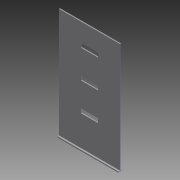
# Autodesk Inventor part: feederStationSlots
Saved by Autodesk Inventor 2011 SP1 (Build 150282100, 282)
## iProperties
Created: 2013-01-18
Part Number: feederStationSlots
Document SubType Name: Modeling
Designer: wes
Density: 1 g/cm^3
Author: wes
Autodesk Inventor part; units mm, degrees
ref_plane "YZ Plane" through (0, 0, 0) normal (1, 0, 0) x (0, 1, 0)
ref_plane "XZ Plane" through (0, 0, 0) normal (0, 1, 0) x (-1, 0, 0)
ref_plane "XY Plane" through (0, 0, 0) normal (0, 0, 1) x (1, 0, 0)
sketch "Sketch1" plane through (0, 0, 0) normal (0, 0, 1) x (1, 0, 0)
  line L0 (-140.3442, -2139.338) -> (951.8558, -2139.338)
  line L1 (951.8558, -2139.338) -> (951.8558, -158.138)
  line L2 (951.8558, -158.138) -> (-140.3442, -158.138)
  line L3 (-140.3442, -158.138) -> (-140.3442, -2139.338)
  line L4 (253.3558, -488.338) -> (558.1558, -488.338)
  line L5 (558.1558, -488.338) -> (558.1558, -564.538)
  line L6 (558.1558, -564.538) -> (253.3558, -564.538)
  line L7 (253.3558, -564.538) -> (253.3558, -488.338)
  line L8 (253.3558, -996.338) -> (558.1558, -996.338)
  line L9 (558.1558, -996.338) -> (558.1558, -1072.538)
  line L10 (558.1558, -1072.538) -> (253.3558, -1072.538)
  line L11 (253.3558, -1072.538) -> (253.3558, -996.338)
  line L12 (253.3558, -1504.338) -> (558.1558, -1504.338)
  line L13 (558.1558, -1504.338) -> (558.1558, -1580.538)
  line L14 (558.1558, -1580.538) -> (253.3558, -1580.538)
  line L15 (253.3558, -1580.538) -> (253.3558, -1504.338)
  point P0 (0, 0)
  dimension "d0" = 1092.2
  dimension "d1" = 1981.2
  dimension "d2" = 393.7
  dimension "d3" = 393.7
  dimension "d4" = 393.7
  dimension "d5" = 304.8
  dimension "d6" = 304.8
  dimension "d7" = 304.8
  dimension "d8" = 76.2
  dimension "d9" = 76.2
  dimension "d10" = 76.2
  dimension "d11" = 558.8
  dimension "d12" = 1066.8
  dimension "d13" = 1574.8
  constraints: 32 end point, 8 parallel, 4 horizontal, 4 perpendicular
  measures "d0" distance of L1.end L2.end
  measures "d1" distance of L2.end L0.start
  measures "d2" distance between parallel lines of L3 L7
  measures "d3" distance between parallel lines of L3 L11
  measures "d4" distance between parallel lines of L3 L15
  measures "d5" distance of L4.start L4.end
  measures "d6" distance of L8.start L8.end
  measures "d7" distance of L12.start L12.end
  measures "d8" distance of L4.end L5.end
  measures "d9" distance of L8.end L9.end
  measures "d10" distance of L12.end L13.end
  measures "d11" distance between parallel lines of L0 L14
  measures "d12" distance between parallel lines of L0 L10
  measures "d13" distance between parallel lines of L0 L6
extrude "Extrusion1" add sketch "Sketch1" against normal blind 19.05
sketch "Sketch2" plane through (-140.3442, -2139.338, 0) normal (0, -1, 0) x (1, 0, 0)
  line L0 (0, -19.05) -> (1092.2, -19.05) projected
  line L1 (1092.2, 0) -> (1092.2, -19.05) projected
  line L2 (0, 0) -> (1092.2, 0) projected
  line L3 (0, 0) -> (0, -19.05) projected
  line L4 (0, -19.05) -> (1092.2, -19.05) projected
  line L5 (1092.2, 0) -> (1092.2, -19.05) projected
  line L6 (0, 0) -> (1092.2, 0) projected
  line L7 (0, 0) -> (0, -19.05) projected
  line L8 (1092.2, 28.575) -> (0, 28.575)
  line L9 (0, 28.575) -> (0, -47.625)
  line L10 (0, -47.625) -> (1092.2, -47.625)
  line L11 (1092.2, -47.625) -> (1092.2, 28.575)
  point P0 (140.3442, 0)
  dimension "d16" = 76.2
  dimension "d17" = 28.575
  constraints: 8 end point, 2 parallel, 1 horizontal, 1 perpendicular
  measures "d16" distance of L10.end L8.start
  measures "d17" distance between parallel lines of L8 L2
extrude "Extrusion2" add sketch "Sketch2" against normal blind 19.05 contours L0 L11 L10 L9 | L9 L8 L11 L2
sketch "Sketch3" plane through (0, 0, -19.05) normal (0, 0, -1) x (-1, 0, 0)
  line L0 (-253.3558, -996.338) -> (-253.3558, -1072.538) projected
  line L1 (-253.3558, -1072.538) -> (-558.1558, -1072.538) projected
  line L2 (-558.1558, -1072.538) -> (-558.1558, -996.338) projected
  line L3 (-253.3558, -488.338) -> (-253.3558, -564.538) projected
  line L4 (-253.3558, -564.538) -> (-558.1558, -564.538) projected
  line L5 (-558.1558, -564.538) -> (-558.1558, -488.338) projected
  line L6 (-253.3558, -1504.338) -> (-253.3558, -1580.538) projected
  line L7 (-253.3558, -1580.538) -> (-558.1558, -1580.538) projected
  line L8 (-558.1558, -1580.538) -> (-558.1558, -1504.338) projected
  point P0 (0, 0)
  point P1 (-507.3558, -589.938)
  point P2 (-304.1558, -589.938)
  point P3 (-507.3558, -1097.938)
  point P4 (-304.1558, -1097.938)
  point P5 (-507.3558, -1605.938)
  point P6 (-304.1558, -1605.938)
  dimension "d20" = 50.8
  dimension "d21" = 50.8
  dimension "d22" = 25.4
  dimension "d23" = 25.4
  dimension "d24" = 50.8
  dimension "d25" = 50.8
  dimension "d26" = 25.4
  dimension "d27" = 25.4
  dimension "d28" = 50.8
  dimension "d29" = 25.4
  dimension "d30" = 50.8
  dimension "d31" = 25.4
  measures "d20" distance from line of point (-507.356, -589.938) L5
  measures "d21" distance from line of point (-304.156, -589.938) L3
  measures "d22" distance from line of point (-304.156, -589.938) L4
  measures "d23" distance from line of L4 point (-507.356, -589.938)
  measures "d24" distance from line of L2 point (-507.356, -1097.938)
  measures "d25" distance from line of L0 point (-304.156, -1097.938)
  measures "d26" distance from line of point (-304.156, -1097.938) L1
  measures "d27" distance from line of L1 point (-507.356, -1097.938)
  measures "d28" distance from line of point (-507.356, -1605.938) L8
  measures "d29" distance from line of L7 point (-507.356, -1605.938)
  measures "d30" distance from line of L6 point (-304.156, -1605.938)
  measures "d31" distance from line of L7 point (-304.156, -1605.938)
hole "Hole1" at (507.3558, -589.938, -19.05) at (304.1558, -589.938, -19.05) at (507.3558, -1097.938, -19.05) at (304.1558, -1097.938, -19.05) at (507.3558, -1605.938, -19.05) at (304.1558, -1605.938, -19.05) direction (0, 0, 1) diameter 6.858 depth 25.4 tip angle 118
thread "Thread1" size "5/16-18 UNC" class "2B" standard "ANSI Unified Screw Threads" full length
thread "Thread2" size "5/16-18 UNC" class "2B" standard "ANSI Unified Screw Threads" full length
thread "Thread3" size "5/16-18 UNC" class "2B" standard "ANSI Unified Screw Threads" full length
thread "Thread4" size "5/16-18 UNC" class "2B" standard "ANSI Unified Screw Threads" full length
thread "Thread5" size "5/16-18 UNC" class "2B" standard "ANSI Unified Screw Threads" full length
thread "Thread6" size "5/16-18 UNC" class "2B" standard "ANSI Unified Screw Threads" full length
equation "\"d6\" = d5"
equation "\"d7\" = d5"
equation "\"d9\" = d8"
equation "\"d10\" = d8"
body "Solid1"
